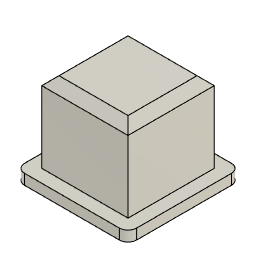
button-cap (Autodesk Fusion 360 design; units mm, degrees)
Autodesk Fusion 360 part; units mm, degrees
note: some values were not read from the file. Set by a fixed rule: which face or edge a step refers to.
sketch "Sketch1" plane through (0, 0, 0) normal (0, 0, 1) x (1, 0, 0)
  line L0 (2.5, -2.5) -> (-2.5, -2.5)
  line L1 (-2.5, -2.5) -> (-2.5, 2.5)
  line L2 (-2.5, 2.5) -> (2.5, 2.5)
  line L3 (2.5, 2.5) -> (2.5, -2.5)
  line L4 (2.5, -2.5) -> (-2.5, 2.5) construction
  line L5 (-2.5, -2.5) -> (2.5, 2.5) construction
  dimension "d1" = 5
  dimension "d2" = 5
  constraint horizontal L0
  constraint perpendicular L0 L1
  constraint parallel L0 L2
  constraint parallel L1 L3
  constraint coincident L4 origin
  constraint coincident L5 origin
  measures "d1" distance of L1.end L2.end
  measures "d2" distance of L0.end L1.end
extrude "Extrude1" add sketch "Sketch1" along normal blind 4.5
chamfer "Chamfer1" distance 0.5 angle 45 4 edges at (0, -2.5, 4.5) (-2.5, 0, 4.5) (0, 2.5, 4.5) (2.5, 0, 4.5)
sketch "Sketch2" plane through (0, 0, 0) normal (0, 0, -1) x (1, 0, 0)
  line L0 (-2.5, -2.5) -> (2.5, -2.5)
  line L1 (2.5, -2.5) -> (2.5, 2.5)
  line L2 (2.5, 2.5) -> (-2.5, 2.5)
  line L3 (-2.5, 2.5) -> (-2.5, -2.5)
  line L4 (1.5, 1.5) -> (-1.5, 1.5)
  line L5 (-1.5, 1.5) -> (-1.5, -1.5)
  line L6 (-1.5, -1.5) -> (1.5, -1.5)
  line L7 (1.5, -1.5) -> (1.5, 1.5)
  line L8 (1.5, 1.5) -> (-1.5, -1.5) construction
  line L9 (-1.5, 1.5) -> (1.5, -1.5) construction
  dimension "d6" = 3
  dimension "d7" = 3
  constraint horizontal L4
  constraint perpendicular L4 L5
  constraint parallel L4 L6
  constraint parallel L5 L7
  constraint coincident L8 origin
  constraint coincident L9 origin
  measures "d6" distance of L5.end L6.end
  measures "d7" distance of L4.end L5.end
extrude "Extrude2" cut sketch "Sketch2" against normal blind 2.75 contours L4 L5 L6 L7
sketch "Sketch4" plane through (0, 0, 0) normal (0, 0, -1) x (1, 0, 0)
  line L0 (-1.5, 1.5) -> (1.5, 1.5)
  line L1 (1.5, 1.5) -> (1.5, -1.5)
  line L2 (1.5, -1.5) -> (-1.5, -1.5)
  line L3 (-1.5, -1.5) -> (-1.5, 1.5)
  line L4 (-2.5, -2.5) -> (2.5, -2.5)
  line L5 (2.5, -2.5) -> (2.5, 2.5)
  line L6 (2.5, 2.5) -> (-2.5, 2.5)
  line L7 (-2.5, 2.5) -> (-2.5, -2.5)
  circle A0 centre (0, 0) radius 2.1213
  constraint coincident A0.centre origin
  constraint coincident L1.end A0
extrude "Extrude4" cut sketch "Sketch4" against normal blind 0.3 contours L0 A0 | L3 A0 | L1 A0 | L2 A0
sketch "Sketch3" plane through (0, 0, 0) normal (0, 0, -1) x (1, 0, 0)
  line L0 (-2.5, -2.5) -> (2.5, -2.5)
  line L1 (2.5, -2.5) -> (2.5, 2.5)
  line L2 (2.5, 2.5) -> (-2.5, 2.5)
  line L3 (-2.5, 2.5) -> (-2.5, -2.5)
  line L4 (3.25, -3.25) -> (-3.25, -3.25)
  line L5 (-3.25, -3.25) -> (-3.25, 3.25)
  line L6 (-3.25, 3.25) -> (3.25, 3.25)
  line L7 (3.25, 3.25) -> (3.25, -3.25)
  line L8 (3.25, -3.25) -> (-3.25, 3.25) construction
  line L9 (-3.25, -3.25) -> (3.25, 3.25) construction
  circle A0 centre (0, 0) radius 2.1213
  dimension "d10" = 6.5
  dimension "d11" = 6.5
  constraint horizontal L4
  constraint perpendicular L4 L5
  constraint parallel L4 L6
  constraint parallel L5 L7
  constraint coincident L8 A0.centre
  constraint coincident L9 A0.centre
  constraint coincident A0.centre origin
  measures "d10" distance of L5.end L6.end
  measures "d11" distance of L4.end L5.end
extrude "Extrude3" add sketch "Sketch3" along normal blind 0.5 contours L0 L1 L2 L3 | L4 L5 L6 L7
fillet "Fillet1" radius 0.5 4 edges at (3.25, -3.25, -0.25) (-3.25, -3.25, -0.25) (3.25, 3.25, -0.25) (-3.25, 3.25, -0.25)
chamfer "Chamfer2" distance 0.2 angle 45 4 edges at (0, -1.5, 2.75) (1.5, 0, 2.75) (0, 1.5, 2.75) (-1.5, 0, 2.75)
move_face "OffsetFaces1" offset -0.15 1 faces at (3, -0.8333, 0)
extrude "Extrude5" add 13 faces at (0.0528, -2.3718, -0.5) (0.7505, 2.7625, -0.5) (-2.4474, 2.4166, -0.5) (-2.7625, -0.7505, -0.5) (-2.4474, -2.4166, -0.5) (0.7505, -2.7375, -0.5) (2.4166, -2.4474, -0.5) (2.7375, -0.7505, -0.5) (2.4166, 2.4474, -0.5) (-2.8376, 2.8208, -0.5) (2.8208, 2.8376, -0.5) (-2.8376, -2.8208, -0.5) (2.8208, -2.8376, -0.5) along direction (0, 0, -1) blind 0.25
sketch "Sketch5" plane through (0, 0, -0.75) normal (0, 0, -1) x (1, 0, 0)
  arc A0 (-3.25, -2.75) -> (-2.75, -3.25) centre (-2.75, -2.75) ccw
  line L0 (-2.75, -3.25) -> (2.75, -3.25)
  arc A1 (2.75, -3.25) -> (3.25, -2.75) centre (2.75, -2.75) ccw
  line L1 (3.25, -2.75) -> (3.25, 2.75)
  arc A2 (3.25, 2.75) -> (2.75, 3.25) centre (2.75, 2.75) ccw
  line L2 (2.75, 3.25) -> (-2.75, 3.25)
  arc A3 (-2.75, 3.25) -> (-3.25, 2.75) centre (-2.75, 2.75) ccw
  line L3 (-3.25, 2.75) -> (-3.25, -2.75)
  circle A4 centre (0, 0) radius 2.1213
  line L4 (2.2, -2.2) -> (-2.2, -2.2) construction
  line L5 (-2.2, -2.2) -> (-2.2, 2.2) construction
  line L6 (-2.2, 2.2) -> (2.2, 2.2) construction
  line L7 (2.2, 2.2) -> (2.2, -2.2) construction
  line L8 (2.2, -2.2) -> (-2.2, 2.2) construction
  line L9 (-2.2, -2.2) -> (2.2, 2.2) construction
  circle A5 centre (2.2, 2.2) radius 0.375 construction
  circle A6 centre (-2.2, 2.2) radius 0.375 construction
  circle A7 centre (-2.2, -2.2) radius 0.375 construction
  circle A8 centre (2.2, -2.2) radius 0.375 construction
  circle A9 centre (2.2, 2.2) radius 0.6
  circle A10 centre (-2.2, 2.2) radius 0.6
  circle A11 centre (-2.2, -2.2) radius 0.6
  circle A12 centre (2.2, -2.2) radius 0.6
  dimension "d22" = 4.4
  dimension "d23" = 4.4
  dimension "d24" = 0.75
  dimension "d25" = 1.2
  constraint horizontal L4
  constraint perpendicular L4 L5
  constraint parallel L4 L6
  constraint parallel L5 L7
  constraint coincident L8 A4.centre
  constraint coincident L9 A4.centre
  constraint coincident A4.centre origin
  constraint coincident L6.end L7.start
  constraint coincident L5.end L6.start
  constraint coincident L4.end L5.start
  constraint coincident L4.start L7.end
  constraint equal A5 A6
  constraint equal A6 A7
  constraint equal A7 A8
  constraint concentric A6 A10
  constraint equal A9 A10
  constraint equal A10 A11
  constraint equal A11 A12
  measures "d22" distance of L5.end L6.end
  measures "d23" distance of L4.end L5.end
  measures "d24" diameter of A5
  measures "d25" diameter of A9
extrude "Extrude6" cut sketch "Sketch5" against normal blind 0.5 contours A9 | A10 | A11 | A12
